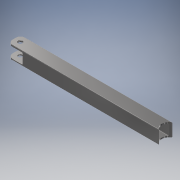
# Autodesk Inventor part: virsutinis
Saved by Autodesk Inventor 2019 (Build 230136000, 136)
## iProperties
Created: 2014-11-18
Part Number: virsutinis
Material: Stainless Steel
Document SubType Name: Modeling
Designer: Ben
Density: 8.08 g/cm^3
Appearance: Semi-Polished
Mass: 2012.63 g
Surface Area: 1247.9 cm^2
Volume: 249.088 cm^3
Author: Ben
Autodesk Inventor part; units mm, degrees
ref_plane "YZ Plane" through (0, 0, 0) normal (1, 0, 0) x (0, 1, 0)
ref_plane "XZ Plane" through (0, 0, 0) normal (0, 1, 0) x (-1, 0, 0)
ref_plane "XY Plane" through (0, 0, 0) normal (0, 0, 1) x (1, 0, 0)
sketch "Sketch1" plane through (0, 0, 0) normal (0, 0, 1) x (1, 0, 0)
  circle A0 centre (0, 0) radius 6
  circle A1 centre (450, 0) radius 11
  line L0 (-3, 20) -> (450, 20)
  line L1 (450, -20) -> (-3, -20)
  line L2 (-18, -5) -> (-18, 5)
  arc A2 (-3, 20) -> (-18, 5) centre (-3, 5) ccw
  arc A3 (-18, -5) -> (-3, -20) centre (-3, -5) ccw
  line L3 (470, 0) -> (470, 0)
  arc A4 (470, 0) -> (450, 20) centre (450, 0) ccw
  arc A5 (450, -20) -> (470, 0) centre (450, 0) ccw
  point P0 (470, -20)
  point P1 (470, 20)
  dimension "d0" = 12
  dimension "d1" = 22
  dimension "d2" = 450
  dimension "d3" = 18
  dimension "d5" = 40
  dimension "d6" = 20
  dimension "d7" = 15
  dimension "d15" = 20
  dimension "d21" = 20
  constraints: 8 end point, 8 point on circle, 8 tangent, 6 centre point, 4 point on line, 2 equal radius, 2 parallel, 1 coincident, 1 horizontal, 1 horizontal alignment, 1 vertical
  measures "d0" diameter of A0
  measures "d1" diameter of A1
  measures "d2" distance of A1.centre A0.centre
  measures "d3" distance from line of L2 point (0, 0)
  measures "d5" distance between parallel lines of L1 L0
  measures "d6" distance from line of L0 A0.centre
  measures "d7" radius of A2
  measures "d15" distance from line of L3 A1.centre
  measures "d21" radius of A4
extrude "Extrusion1" add sketch "Sketch1" along normal blind 40
ref_plane "Work Plane1" through (0, 0, 20) normal (0, 0, 1) x (1, 0, 0)
chamfer "Chamfer1" distance 1 angle 45 2 edges at (-6, 0, 0) (-6, 0, 40)
body "Solid1"
